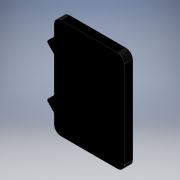
# Autodesk Inventor part: SCHUNK-9962713 Bracket MPG 40
Saved by Autodesk Inventor 2019 (Build 230136000, 136)
## iProperties
Created: 2022-08-29
Part Number: SCHUNK-9962713 Bracket MPG 40
Material: Generic
Catalog Web Link: www.cadenas.de
Description: holder-MPG
Vendor: SCHUNK
Document SubType Name: Modeling
Designer: psAdmin
Manufacturer: SCHUNK
Mass: 0.0998269 g
Surface Area: 2.39965 cm^2
Volume: 0.0998269 cm^3
Density: 1 g/cm^3
Appearance: PSOLRGB-128-128-128
Category: PARTsolutions
Company: SCHUNK
Title: SCHUNK-9962713 Bracket MPG 40
Author: Cadenas PARTsolutions
Comments: MPG
PSOL_IDENT_0: {$CADENAS_DATA/23d-libs/schunk/greifsysteme/greifmodule/greifmodule_pneumatisch/2_finger_parallelgre
PSOL_IDENT_1: ifer/2_finger_kleinteilegreifer/mpg/mpg_hal.prj},198 {VTYP=3D},{NB=SCHUNK-9962713 Bracket MPG 40},{L
PSOL_IDENT_2: INA=SCHUNK-9962713 Bracket MPG 40},{NN=holder},{DATE=22.12.2021 07:16:22},{GEOMDATE=15.04.2020 08:38
PSOL_IDENT_3: :32},{VERSION=},{LINEID=70},{WBVAR=},{WBNUMERIC=}  {NB=SCHUNK-9962713 Halter MPG 40},{LINA=SCHUNK-99
PSOL_IDENT_4: 62713 Halter MPG 40},{KT=DUMMY},{IDNR=9962713},{TYP=MPG 40},{TYP1=7.000},{TYP2=2.000},{B=9.200},{B1=
PSOL_IDENT_5: 8.300},{B2=3.800},{H=11.900},{H1=6.000},{H2=6.000},{D1=2.800},{L1=4.400},{H4=1.000},{H3=2.000},{DSA=
PSOL_IDENT_6: 5.500},{HS=1.000},{DSI=3.100},{CNSCTN=84799070}
NB: SCHUNK-9962713 Bracket MPG 40
NN: holder
NT: MPG
NBSYN: SCHUNK-$IDNR. Bracket $TYP.
LINA: SCHUNK-9962713 Bracket MPG 40
CATALOG: SCHUNK
IDNR: 9962713
TYP: MPG 40
TYP1: 7
TYP2: 2
B: 9.2
B1: 8.3
B2: 3.8
H: 11.9
H1: 6
H2: 6
D1: 2.8
L1: 4.4
H4: 1
H3: 2
DSA: 5.5
HS: 1
DSI: 3.1
CNSCTN: 84799070
SUPPLIER: SCHUNK
ARTICLENO: SCHUNK-9962713 Bracket MPG 40
BOMINFO: SCHUNK-9962713 Bracket MPG 40
CREATOR: CADENAS GmbH
Autodesk Inventor part; units mm, degrees
sketch "Sketch_1" plane through (0, 0, 0) normal (0, 0, 1) x (1, 0, 0)
  arc A0 (-5.2586, 3.1414) -> (-5.2586, 2.8586) centre (-5.1172, 3) ccw
  line L0 (-5.2586, 2.8586) -> (-4.5586, 2.1586)
  arc A1 (-4.5, 2.0172) -> (-4.5586, 2.1586) centre (-4.7, 2.0172) ccw
  line L1 (-4.5, 2.0172) -> (-4.5, -2.0172)
  arc A2 (-4.5586, -2.1586) -> (-4.5, -2.0172) centre (-4.7, -2.0172) ccw
  line L2 (-4.5586, -2.1586) -> (-5.2586, -2.8586)
  arc A3 (-5.2586, -2.8586) -> (-5.2586, -3.1414) centre (-5.1172, -3) ccw
  line L3 (-5.2586, -3.1414) -> (-4.5586, -3.8414)
  arc A4 (-4.5, -3.9828) -> (-4.5586, -3.8414) centre (-4.7, -3.9828) ccw
  line L4 (-4.5, -3.9828) -> (-4.5, -5.1)
  arc A5 (-4.5, -5.1) -> (-3.7, -5.9) centre (-3.7, -5.1) ccw
  line L5 (-3.7, -5.9) -> (3, -5.9)
  arc A6 (3, -5.9) -> (3.8, -5.1) centre (3, -5.1) ccw
  line L6 (3.8, -5.1) -> (3.8, 5.2)
  arc A7 (3.8, 5.2) -> (3, 6) centre (3, 5.2) ccw
  line L7 (3, 6) -> (-3.7, 6)
  arc A8 (-3.7, 6) -> (-4.5, 5.2) centre (-3.7, 5.2) ccw
  line L8 (-4.5, 5.2) -> (-4.5, 3.9828)
  arc A9 (-4.5586, 3.8414) -> (-4.5, 3.9828) centre (-4.7, 3.9828) ccw
  line L9 (-4.5586, 3.8414) -> (-5.2586, 3.1414)
  constraints: 20 end point, 20 point on circle, 10 centre point
extrude "Extrusion1" add sketch "Sketch_1" along normal blind 1
ref_plane "hal_XY" through (0, 0, 0) normal (0, 0, 1) x (1, 0, 0)
ref_plane "hal_YZ" through (0, 0, 0) normal (1, 0, 0) x (0, 1, 0)
ref_plane "hal_ZX" through (0, 0, 0) normal (0, 1, 0) x (0, 0, 1)
ref_plane "s01_XY" through (0, 0, 1) normal (0, 0, 1) x (1, 0, 0)
ref_plane "s01_YZ" through (0, 0, 1) normal (1, 0, 0) x (0, 1, 0)
ref_plane "s01_ZX" through (0, 0, 1) normal (0, 1, 0) x (0, 0, 1)
body "Solid1"
